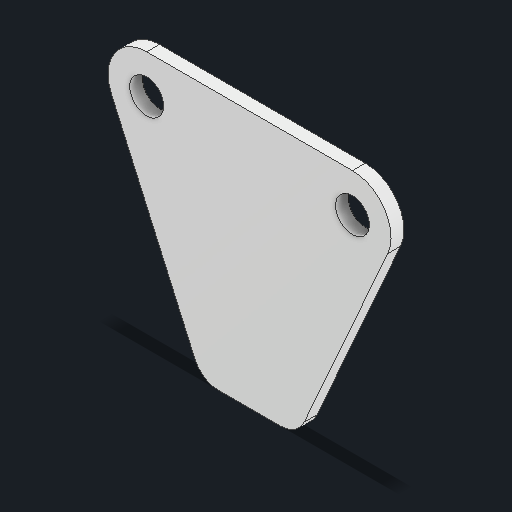
# Autodesk Inventor part: Flap Gusset
Saved by Autodesk Inventor 2025.1 (Build 291241000, 241)
## iProperties
Created: 2024-10-13
Part Number: Flap Gusset
Material: Acetal Resin, White
Document SubType Name: Sheet Metal
Designer: Averey Ku
Density: 1.425 g/cm^3
Appearance: Smooth - White
Flat Pattern Width: 3.38467 cm
Flat Pattern Length: 3.55082 cm
Flat Pattern Area: 12.0183 cm^2
Sheet Metal Rule: Default_mm
Sheet Metal Width: 1.333 in
Sheet Metal Length: 1.398 in
Sheet Metal Area: 1.863 in^2
Author: Averey Ku
Autodesk Inventor part; units mm, degrees
ref_plane "YZ Plane" through (0, 0, 0) normal (1, 0, 0) x (0, 1, 0)
ref_plane "XZ Plane" through (0, 0, 0) normal (0, 1, 0) x (-1, 0, 0)
ref_plane "XY Plane" through (0, 0, 0) normal (0, 0, 1) x (1, 0, 0)
sketch "Sketch1" plane through (0, 0, 0) normal (0, 0, 1) x (1, 0, 0)
  circle A0 centre (13.2036, 20.3187) radius 2.0955
  circle A1 centre (-12.1964, 20.3187) radius 2.0955
  line L0 (4.3471, -6.6688) -> (-3.3398, -6.6688)
  arc A2 (4.3471, -6.6688) -> (7.3873, -4.4091) centre (4.3471, -3.4938) ccw
  arc A3 (-6.38, -4.4091) -> (-3.3398, -6.6688) centre (-3.3398, -3.4938) ccw
  line L1 (-16.5477, 18.3828) -> (-6.2406, -4.7844)
  line L2 (17.5549, 18.3828) -> (7.2479, -4.7844)
  arc A4 (-12.1964, 25.0812) -> (-16.5477, 18.3828) centre (-12.1964, 20.3187) ccw
  arc A5 (17.5549, 18.3828) -> (13.2036, 25.0812) centre (13.2036, 20.3187) ccw
  line L3 (-12.1964, 25.0812) -> (13.2036, 25.0812)
  point P0 (0, 0)
  point P1 (-12.1964, 25.0812)
  point P2 (17.4758, 18.214)
  point P3 (-16.4686, 18.214)
  dimension "d1" = 3.175
  dimension "d8" = 4.191
  dimension "d9" = 4.191
  dimension "d25" = 9.525
  dimension "d26" = 9.525
  dimension "d28" = 31.75
  constraints: 10 point on circle, 8 end point, 7 tangent, 6 centre point, 2 coincident, 1 equal radius, 1 horizontal, 2 other
  measures "d1" radius of A2
  measures "d8" diameter of A1
  measures "d9" diameter of A0
  measures "d25" diameter of A4
  measures "d26" diameter of A5
  measures "d28" distance between parallel lines of L0 L3
extrude "Extrusion1" add sketch "Sketch1" along normal blind 1.5875
equation "\"BendRadius\" = Thickness"
equation "\"BendReliefWidth\" = Thickness"
equation "\"BendReliefDepth\" = 0.5 * Thickness"
equation "\"CornerReliefSize\" = 4 * Thickness"
equation "\"MinimumRemnant\" = 2 * Thickness"
equation "\"TransitionRadius\" = BendRadius"
equation "\"JacobiRadiusSize\" = BendRadius"
equation "\"GapSize\" = Thickness"
equation "\"Thickness\" = 1.5875"
body "Solid1"
